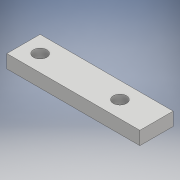
# Autodesk Inventor part: plaque 1
Saved by Autodesk Inventor 2018.1 (Build 221171000, 171)
## iProperties
Created: 2022-06-29
Part Number: plaque 1
Material: Generic
Document SubType Name: Modeling
Designer: Bureau
Density: 1 g/cm^3
Appearance: Default
Author: Bureau
Autodesk Inventor part; units mm, degrees
ref_plane "YZ Plane" through (0, 0, 0) normal (1, 0, 0) x (0, 1, 0)
ref_plane "XZ Plane" through (0, 0, 0) normal (0, 1, 0) x (-1, 0, 0)
ref_plane "XY Plane" through (0, 0, 0) normal (0, 0, 1) x (1, 0, 0)
sketch "Sketch1" plane through (0, 0, 0) normal (0, 0, 1) x (1, 0, 0)
  circle A0 centre (0, 0) radius 4
  line L0 (0, 0) -> (48, 0)
  circle A1 centre (48, 0) radius 4
  line L1 (0, 0) -> (0, 10)
  line L2 (0, 10) -> (70, 10)
  line L3 (70, 10) -> (70, -10)
  line L4 (70, -10) -> (-10, -10)
  line L5 (-10, -10) -> (-10, 10)
  line L6 (-10, 10) -> (0, 10)
  dimension "d0" = 8
  dimension "d1" = 48
  dimension "d2" = 8
  dimension "d3" = 10
  dimension "d4" = 70
  dimension "d5" = 20
  dimension "d6" = 80
  constraints: 14 end point, 5 perpendicular, 2 centre point, 2 coincident, 1 horizontal, 1 point on line, 1 vertical
  measures "d0" diameter of A0
  measures "d1" distance of L0.start L0.end
  measures "d2" diameter of A1
  measures "d3" distance of L0.start L1.end
  measures "d4" distance of L1.end L2.end
  measures "d5" distance of L2.end L3.end
  measures "d6" distance of L3.end L4.end
extrude "Extrusion1" add sketch "Sketch1" along normal blind 8
body "Solid1"
